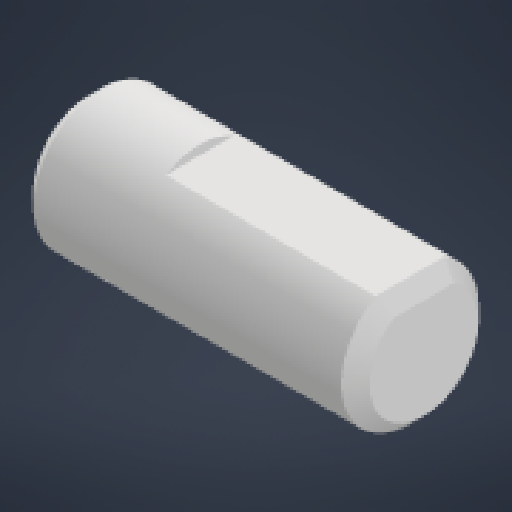
# Autodesk Inventor part: parrallelShaftPin
Saved by Autodesk Inventor 2026.3 (Build 303398000, 398)
## iProperties
Created: 2026-05-02
Part Number: parrallelShaftPin
Material: Generic
Document SubType Name: Modeling
Designer: frede
Density: 1 g/cm^3
Appearance: Default
Author: frede
Autodesk Inventor part; units mm, degrees
ref_plane "YZ Plane" through (0, 0, 0) normal (1, 0, 0) x (0, 1, 0)
ref_plane "XZ Plane" through (0, 0, 0) normal (0, 1, 0) x (-1, 0, 0)
ref_plane "XY Plane" through (0, 0, 0) normal (0, 0, 1) x (1, 0, 0)
sketch "Sketch1" plane through (0, 0, 0) normal (1, 0, 0) x (0, 1, 0)
  circle A0 centre (0, 0) radius 2.45
  dimension "d0" = 4.9
  constraints: 1 centre point, 1 coincident
  measures "d0" diameter of A0
extrude "Extrusion1" add sketch "Sketch1" along normal blind 15
sketch "Sketch2" plane through (15, 0, 0) normal (1, 0, 0) x (0, 0, -1)
  circle A0 centre (0, 0) radius 2.45 projected
  line L0 (-1.228, 2.12) -> (1.228, 2.12)
  dimension "d6" = 0.33
  constraints: 2 end point, 2 point on circle, 1 horizontal
  measures "d6" distance edge to line of A0 L0
extrude "Extrusion2" cut sketch "Sketch2" against normal blind 8 contours L0 A0 picked at (-0.0856, 2.2255)
chamfer "Chamfer1" distance 0.5 angle 45 3 edges at (15, -2.45, 0) (0, -2.45, 0) (15, 2.12, 0)
body "Solid1"
